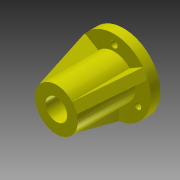
# Autodesk Inventor part: GUIDE
Saved by Autodesk Inventor 2013 (Build 170138000, 138)
## iProperties
Created: 2013-12-05
Part Number: GUIDE
Material: Generic
Document SubType Name: Modeling
Designer: employee
Density: 1 g/cm^3
Author: employee
Autodesk Inventor part; units mm, degrees
ref_plane "YZ Plane" through (0, 0, 0) normal (1, 0, 0) x (0, 1, 0)
ref_plane "XZ Plane" through (0, 0, 0) normal (0, 1, 0) x (-1, 0, 0)
ref_plane "XY Plane" through (0, 0, 0) normal (0, 0, 1) x (1, 0, 0)
sketch "Sketch1" plane through (0, 0, 0) normal (0, 0, 1) x (1, 0, 0)
  circle A0 centre (0, 0) radius 19.05
  circle A1 centre (0, 0) radius 5.6063
  dimension "d0" = 11.2125
  dimension "d2" = 38.1
  constraints: 2 centre point, 2 coincident
  measures "d0" diameter of A1
  measures "d2" diameter of A0
extrude "Extrusion1" add sketch "Sketch1" along normal blind 5
sketch "Sketch2" plane through (0, 0, 5) normal (0, 0, 1) x (1, 0, 0)
  circle A0 centre (0, 0) radius 5.6063 projected
  circle A1 centre (0, 0) radius 19.05 projected
  circle A2 centre (0, 0) radius 14.2875
  circle A3 centre (0, 0) radius 11.1125
  dimension "d5" = 28.575
  dimension "d26" = 22.225
  constraints: 2 centre point, 2 coincident
  measures "d5" diameter of A2
  measures "d26" diameter of A3
extrude "Extrusion2" add sketch "Sketch2" along normal blind 30 contours A3
sketch "Sketch3" plane through (0, 0, 5) normal (0, 0, 1) x (1, 0, 0)
  circle A0 centre (0, 0) radius 11.1125 projected
  circle A1 centre (0, 14.2875) radius 1.75
  dimension "d11" = 14.2875
  dimension "d12" = 3.5
  constraints: 1 centre point, 1 vertical alignment
  measures "d11" distance of A1.centre A0.centre
  measures "d12" diameter of A1
extrude "Extrusion3" cut sketch "Sketch3" against normal through all contours A1
sketch "Sketch4" plane through (0, 0, 0) normal (1, 0, 0) x (0, 1, 0)
  line L0 (11.1125, 35) -> (11.1125, 5) projected
  line L1 (11.1125, 5) -> (12.5375, 5) projected
  line L2 (12.5375, 5) -> (12.5375, 0) projected
  line L3 (12.5375, 0) -> (5.6063, 0) projected
  line L4 (5.6063, 0) -> (5.6063, 35) projected
  line L5 (5.6063, 35) -> (11.1125, 35) projected
  line L6 (-19.05, 0) -> (-19.05, 5) projected
  line L7 (-19.05, 5) -> (-11.1125, 5) projected
  line L8 (-11.1125, 5) -> (-11.1125, 35) projected
  line L9 (-11.1125, 35) -> (-5.6063, 35) projected
  line L10 (-5.6063, 35) -> (-5.6063, 0) projected
  line L11 (-5.6063, 0) -> (-19.05, 0) projected
  line L12 (19.05, 5) -> (19.05, 0) projected
  line L13 (19.05, 0) -> (16.0375, 0) projected
  line L14 (16.0375, 0) -> (16.0375, 5) projected
  line L15 (16.0375, 5) -> (19.05, 5) projected
  line L16 (-19.05, 5) -> (-11.1125, 5)
  line L17 (-11.1125, 35) -> (-19.05, 5)
  line L18 (-11.1125, 35) -> (-11.1125, 5)
  point P0 (0, 0)
  constraints: 6 end point, 1 collinear, 1 perpendicular
extrude "Extrusion4" add sketch "Sketch4" along normal mid plane 5 contours L17 L8 L7
sketch "Sketch5" plane through (0, 0, 35) normal (0, 0, 1) x (1, 0, 0)
  circle A0 centre (0, 0) radius 11.1125 projected
  line L0 (2.5, -19.05) -> (0, -19.05) projected
  line L1 (2.5, -11.1125) -> (2.5, -19.05) projected
  line L2 (0, -11.1125) -> (2.5, -11.1125) projected
  line L3 (-2.5, -11.1125) -> (0, -11.1125) projected
  line L4 (-2.5, -19.05) -> (-2.5, -11.1125) projected
  line L5 (0, -19.05) -> (-2.5, -19.05) projected
  line L6 (-2.5, -11.1125) -> (2.5, -11.1125)
  line L7 (2.5, -11.1125) -> (2.5, -10.8276)
  line L8 (2.5, -10.8276) -> (-2.5, -10.8276)
  line L9 (-2.5, -10.8276) -> (-2.5, -11.1125)
  constraints: 8 end point, 2 parallel, 1 horizontal, 1 perpendicular, 1 point on circle
extrude "Extrusion5" add sketch "Sketch5" against normal up to surface (30 mm away) contours L8 A0 | A0 L3 L9 | L7 L2 A0 picked at (-0.5582, -10.8803)
sketch "Sketch6" plane through (0, 0, 0) normal (0, 0, -1) x (-1, 0, 0)
  circle A0 centre (0, 0) radius 19.05 projected
  circle A1 centre (0, 0) radius 25.4
  dimension "d19" = 6.35
  constraints: 1 centre point, 1 coincident
  measures "d19" radial gap between concentric circles of A0 A1
extrude "Extrusion6" cut sketch "Sketch6" against normal through all
pattern_circular "Circular Pattern1" count 3 over 360 about axis through (0, 0, 5) along (0, 0, 1) of "Extrusion6", "Extrusion5", "Extrusion4", "Extrusion3"
body "Solid1"
